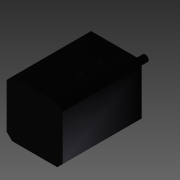
# Autodesk Inventor part: StepperMotorNema17
Saved by Autodesk Inventor 2016 (Build 200138000, 138)
## iProperties
Company: RobotDigg
Category: Electronics
Created: 2013-11-24
Part Number: StepperMotorNema17
Material: Generic
Document SubType Name: Modeling
Designer: Jack
Density: 1 g/cm^3
Appearance: Smooth - Black
Mass: 106.481 g
Surface Area: 137.531 cm^2
Volume: 106.481 cm^3
Vendor: RobotDigg
Catalog Web Link: http://www.robotdigg.com/product/29/Nema17-60mm-1.5A-high-torque-stepper-motor
Author: Jack
Title: NEMA 17 x 60 Stepper Motor
Autodesk Inventor part; units mm, degrees
ref_plane "YZ Plane" through (0, 0, 0) normal (1, 0, 0) x (0, 1, 0)
ref_plane "XZ Plane" through (0, 0, 0) normal (0, 1, 0) x (-1, 0, 0)
ref_plane "XY Plane" through (0, 0, 0) normal (0, 0, 1) x (1, 0, 0)
sketch "Sketch1" plane through (0, 0, 0) normal (0, 1, 0) x (-1, 0, 0)
  line L0 (0, 0) -> (42.3, 0)
  line L1 (42.3, 0) -> (42.3, 42.3)
  line L2 (42.3, 42.3) -> (0, 42.3)
  line L3 (0, 42.3) -> (0, 0)
  dimension "d0" = 42.3
  dimension "d1" = 42.3
  constraints: 8 end point, 2 perpendicular, 1 horizontal, 1 parallel
  measures "d0" distance of L0.start L0.end
  measures "d1" distance of L0.end L1.end
extrude "Extrusion1" add sketch "Sketch1" along normal blind 60
sketch "Sketch2" plane through (0, 60, 0) normal (0, 1, 0) x (1, 0, 0)
  line L0 (0, 0) -> (-42.3, 0) projected
  line L1 (0, -42.3) -> (0, 0) projected
  circle A0 centre (-21.15, -21.15) radius 11
  point P0 (0, -2)
  point P1 (-2, 0)
  point P2 (-40.3, 0)
  point P3 (0, -40.3)
  dimension "d6" = 22
  dimension "d7" = 21.15
  dimension "d8" = 21.15
  constraints: 1 centre point
  measures "d6" diameter of A0
  measures "d7" distance from line of L0 A0.centre
  measures "d8" distance from line of L1 A0.centre
extrude "Extrusion2" add sketch "Sketch2" along normal blind 2
sketch "Sketch3" plane through (-21.15, 62, 21.15) normal (0, 1, 0) x (1, 0, 0)
  circle A0 centre (0, 0) radius 11 projected
  circle A1 centre (0, 0) radius 2.5
  point P0 (21.15, 21.15)
  dimension "d11" = 5
  constraints: 1 centre point, 1 coincident
  measures "d11" diameter of A1
extrude "Extrusion3" add sketch "Sketch3" along normal blind 22 contours A1
sketch "Sketch4" plane through (-21.15, 84, 21.15) normal (0, 1, 0) x (1, 0, 0)
  circle A0 centre (0, 0) radius 2.5 projected
  line L0 (-1.5, 2) -> (1.5, 2)
  point P0 (21.15, 21.15)
  dimension "d14" = 2
  constraints: 2 end point, 2 point on circle, 1 horizontal
  measures "d14" distance from line of A0.centre L0
extrude "Extrusion4" cut sketch "Sketch4" against normal blind 21 contours L0 A0 picked at (-0.3466, 2.0912)
sketch "Sketch5" plane through (0, 60, 0) normal (0, 1, 0) x (1, 0, 0)
  line L0 (-42.3, 0) -> (-42.3, -42.3) projected
  line L1 (-42.3, -42.3) -> (0, -42.3) projected
  circle A0 centre (-36.65, -5.65) radius 1.5
  circle A1 centre (-5.65, -5.65) radius 1.5
  circle A2 centre (-5.65, -36.65) radius 1.5
  circle A3 centre (-36.65, -36.65) radius 1.5
  point P0 (-42.3, -2)
  point P1 (-42.3, -40.3)
  point P2 (-40.3, -42.3)
  point P3 (-2, -42.3)
  point P4 (0, 0)
  dimension "d17" = 3
  dimension "d18" = 3
  dimension "d19" = 3
  dimension "d20" = 3
  dimension "d21" = 31
  dimension "d22" = 5.65
  dimension "d23" = 31
  dimension "d24" = 5.65
  constraints: 4 centre point, 2 horizontal alignment, 2 vertical alignment
  measures "d17" diameter of A0
  measures "d18" diameter of A1
  measures "d19" diameter of A2
  measures "d20" diameter of A3
  measures "d21" distance of A3.centre A0.centre
  measures "d22" distance from line of L1 A3.centre
  measures "d23" distance of A2.centre A3.centre
  measures "d24" distance from line of L0 A3.centre
extrude "Extrusion5" cut sketch "Sketch5" against normal blind 4.5
chamfer "Chamfer1" distance 4 angle 45 4 edges at (-42.3, 30, 0) (-42.3, 30, 42.3) (0, 30, 0) (0, 30, 42.3)
body "Solid1"
